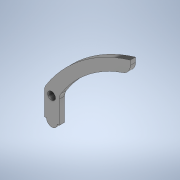
# Autodesk Inventor part: Part59
Saved by Autodesk Inventor 2021 (Build 250183000, 183)
## iProperties
Created: 2020-12-03
Part Number: Part59
Material: Nickel-Copper Alloy 400
Document SubType Name: Modeling
Designer: pedro
Density: 8.83 g/cm^3
Appearance: Cromado - Preto polido
Author: pedro
Autodesk Inventor part; units mm, degrees
ref_plane "YZ Plane" through (0, 0, 0) normal (1, 0, 0) x (0, 1, 0)
ref_plane "XZ Plane" through (0, 0, 0) normal (0, 1, 0) x (-1, 0, 0)
ref_plane "XY Plane" through (0, 0, 0) normal (0, 0, 1) x (1, 0, 0)
sketch "Sketch1" plane through (0, 0, 0) normal (0, 0, 1) x (1, 0, 0)
  circle A0 centre (-0.0549, 4.1489) radius 0.75
  line L0 (-1.4285, -0.0001) -> (-1.4285, 4.899)
  line L1 (-1.4285, 4.899) -> (1.4285, 4.899) construction
  line L2 (1.4285, 4.899) -> (1.4285, 0)
  circle A1 centre (0, 0) radius 1.0285
  line L3 (-1.0285, -0.0001) -> (-1.4285, -0.0001)
  line L4 (1.0285, 0) -> (1.4285, 0)
  line L5 (0, 0) -> (15, 0)
  arc A2 (15, 17.5757) -> (-1.4285, 4.899) centre (23.253, -10.1036) ccw
  arc A3 (15, 15.2472) -> (1.4285, 4.899) centre (21.0936, -6.818) ccw
  line L6 (15, 15.2472) -> (15, 17.5757)
  point P0 (0.0155, 4.8988)
  dimension "d6" = 1.5
  dimension "d28" = 2.057
  dimension "d29" = 0.4
  dimension "d30" = 0.4
  dimension "d33" = 15
  constraints: 14 end point, 6 point on circle, 4 centre point, 3 horizontal, 2 perpendicular, 2 vertical, 1 coincident
  measures "d6" diameter of A0
  measures "d28" diameter of A1
  measures "d29" distance of L4.start L2.end
  measures "d30" distance of L3.start L0.start
  measures "d33" distance of L5.start L5.end
extrude "Extrusion1" add sketch "Sketch1" along normal blind 1 contours L0 A2 L6 A3 L2 L4 A1 L3
extrude "Extrusion2" add sketch "Sketch1" along normal blind 1 contours A1
fillet "Fillet5" radius 2 3 edges at (15, 15.2472, 0.5) (-1.4285, 4.899, 0.5) (1.4285, 4.899, 0.5)
body "Solid1"
